Autodesk Fusion 360 part; units mm, degrees
(part 7 of 7)
  spline S47 degree 3 poles (-28.9778, 7.7644) (-29.036, 7.5424) (-29.0052, 7.3365) (-28.9606, 7.2236) (-28.942, 7.1764) (-28.9203, 7.1406) (-28.9025, 7.1161) (-28.8924, 7.1022) (-28.884, 7.0919) (-28.8332, 7.031) (-28.8015, 6.993) (-28.7553, 6.947) (-28.6638, 6.8038) (-28.5987, 6.7019) (-28.4905, 6.5146) (-28.4393, 6.242) (-28.3991, 6.0278) (-28.4161, 5.8162) (-28.4329, 5.7122) (-28.4484, 5.6167) (-28.4607, 5.5388) (-28.5278, 5.3746) (-28.6119, 5.1689) (-28.789, 4.9345) (-28.9196, 4.8156) (-29.1619, 4.5951) (-29.2503, 4.5799) (-29.3108, 4.5478) (-29.445, 4.4767) (-29.4238, 4.4889) (-29.4531, 4.4677) (-29.5491, 4.3982) (-29.7033, 4.2078) (-29.7434, 3.9157) knots 0.001251 0.001251 0.001251 0.001251 0.25 0.25 0.25 0.35404 0.35404 0.35404 0.412746 0.412746 0.412746 0.449449 0.449449 0.449449 0.475576 0.475576 0.475576 0.496118 0.496118 0.496118 0.514995 0.514995 0.514995 0.538647 0.538647 0.538647 0.582499 0.582499 0.582499 0.679826 0.679826 0.679826 0.99875 0.99875 0.99875 0.99875
  dimension "d71" = 1.5
  dimension "d72" = -1.5
  dimension "d74" = 360
  dimension "d75" = 30
  dimension "d76" = 1.5
  dimension "d77" = -1.5
  dimension "d78" = 60
  dimension "d79" = -3
  dimension "d80" = 3
  dimension "d82" = 360
  constraint coincident A3.centre L0.start
  constraint concentric A6 A9
  measures "d75" diameter of A6
  measures "d78" diameter of A9
extrude "Extrude3" cut sketch "Sketch3" against normal blind 6 contours L5 L8 A7 A10 A13 A14 | L3 L6 A7 A10 A12 A13 | L2 L4 A7 A10 A11 A12 | L7 L10 A7 A10 A14 A15 | L1 L9 A7 A10 A11 A15
fillet "Fillet2" radius 3 30 edges at (9.7572, -25.1753, 1.2) (8.4902, -21.2758, 1.2) (12.0526, -11.2687, 1.2) (14.4417, -7.9805, 1.2) (22.8581, -1.4999, 1.2) (26.9583, -1.4999, 1.2) (6.9041, -26.1024, 1.2) (5.637, -22.2029, 1.2) (-3.1272, -16.2009, 1.2) (-6.9927, -14.945, 1.2) (-17.6109, -14.6492, 1.2) (-20.928, -17.0593, 1.2) (-22.6914, -14.6322, 1.2) (-19.3742, -12.2222, 1.2) (-16.3744, -2.0322, 1.2) (-16.3744, 2.0322, 1.2) (-19.3743, 12.2221, 1.2) (-22.6915, 14.6321, 1.2) (-20.9281, 17.0591, 1.2) (-17.611, 14.6491, 1.2) (-6.9927, 14.945, 1.2) (-3.1272, 16.2009, 1.2) (5.6369, 22.2029, 1.2) (6.9039, 26.1024, 1.2) (9.7571, 25.1754, 1.2) (8.4901, 21.2759, 1.2) (12.0526, 11.2687, 1.2) (14.4417, 7.9805, 1.2) (22.8581, 1.5001, 1.2) (26.9583, 1.5001, 1.2)
mirror "Mirror1" about plane through (0, 0, 0) normal (0, 0, -1) of bodies 1 merged
equation "d1 = ( 30.367 * 2 ) * 1 mm"
equation "d2 = ( 0.633 * 2 ) * 1 mm"
equation "d22 = ( 49 * 0.5 ) * 1 deg"
equation "d27 = ( 49 * 1.5 ) * 1 deg"
equation "d29 = ( 49 * 2 ) * 1 deg"
equation "d32 = ( 49 * 2.5 ) * 1 deg"
equation "d33 = ( 49 * 3 ) * 1 deg"
equation "d35 = ( 49 * 3.5 ) * 1 deg"
equation "d56 = ( 7.5 * 49 ) * 1 deg"
